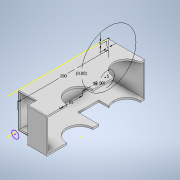
# Autodesk Inventor part: 차체 뚜껑
Saved by Autodesk Inventor 2021 (Build 250183000, 183)
## iProperties
Created: 2022-09-27
Part Number: 차체 뚜껑
Material: 일반
Document SubType Name: Modeling
Designer: SW2151
Density: 1 g/cm^3
Appearance: 기본값
Author: SW2151
Autodesk Inventor part; units mm, degrees
ref_plane "YZ Plane" through (0, 0, 0) normal (1, 0, 0) x (0, 1, 0)
ref_plane "XZ Plane" through (0, 0, 0) normal (0, 1, 0) x (-1, 0, 0)
ref_plane "XY Plane" through (0, 0, 0) normal (0, 0, 1) x (1, 0, 0)
sketch "스케치1" plane through (0, 0, 0) normal (0, 1, 0) x (-1, 0, 0)
  line L0 (4.1347, 105.7038) -> (-100.8653, 105.7038)
  line L1 (-100.8653, 105.7038) -> (-100.8653, -184.2962)
  line L2 (-100.8653, -184.2962) -> (4.1347, -184.2962)
  line L3 (4.1347, -184.2962) -> (4.1347, 105.7038)
  point P0 (0, 0)
  dimension "d0" = 105
  dimension "d1" = 290
  constraints: 8 end point, 2 parallel, 1 horizontal, 1 perpendicular
  measures "d0" distance of L2.end L1.end
  measures "d1" distance of L1.end L0.end
sketch "스케치2" plane through (0, 0, 0) normal (0, 1, 0) x (-1, 0, 0)
  point P0 (0, 0)
sketch "스케치3" plane through (0, 0, 0) normal (0, 1, 0) x (-1, 0, 0)
  point P0 (0, 0)
sketch "스케치4" plane through (0, 0, 0) normal (0, 1, 0) x (-1, 0, 0)
  point P0 (0, 0)
extrude "돌출1" add sketch "스케치1" along normal blind 100
sketch "스케치5" plane through (100.8653, 0, 105.7038) normal (1, 0, 0) x (0, 0, -1)
  line L0 (0, 0) -> (290, 0) projected
  line L1 (290, 0) -> (285, 0)
  line L2 (285, 0) -> (285, 5)
  line L3 (285, 5) -> (290, 5)
  line L4 (290, 5) -> (290, 0)
  line L5 (290, 0) -> (290, 100) projected
  line L6 (290, 100) -> (285, 100)
  line L7 (285, 100) -> (285, 95)
  line L8 (285, 95) -> (290, 95)
  line L9 (290, 95) -> (290, 100)
  line L10 (285, 5) -> (35, 5)
  line L11 (35, 5) -> (35, 95)
  line L12 (35, 95) -> (285, 95)
  line L13 (285, 95) -> (285, 5)
  point P0 (105.7038, 0)
  dimension "d4" = 5
  dimension "d5" = 5
  dimension "d6" = 5
  dimension "d7" = 5
  dimension "d8" = 250
  dimension "d9" = 90
  constraints: 24 end point, 6 parallel, 3 horizontal, 3 perpendicular
  measures "d4" distance of L2.end L3.end
  measures "d5" distance of L1.end L2.end
  measures "d6" distance of L8.end L7.end
  measures "d7" distance of L7.end L6.end
  measures "d8" distance of L11.end L12.end
  measures "d9" distance of L10.end L11.end
extrude "돌출2" cut sketch "스케치5" against normal blind 100 contours L10 L11 L12 L13
sketch "스케치6" plane through (100.8653, 0, 105.7038) normal (1, 0, 0) x (0, 0, -1)
  point P0 (105.7038, 0)
sketch "스케치7" plane through (100.8653, 0, 105.7038) normal (1, 0, 0) x (0, 0, -1)
  line L0 (285, 5) -> (35, 5) projected
  line L1 (35, 5) -> (11, 5)
  line L2 (11, 5) -> (11, 95)
  line L3 (11, 95) -> (35, 95)
  line L4 (35, 95) -> (35, 5)
  point P0 (105.7038, 0)
  dimension "d12" = 24
  constraints: 8 end point, 2 parallel, 1 horizontal, 1 perpendicular
  measures "d12" distance of L2.end L3.end
extrude "돌출3" cut sketch "스케치7" against normal blind 100
sketch "스케치8" plane through (-4.1347, 0, 105.7038) normal (0, 0, 1) x (1, 0, 0)
  circle A0 centre (22.6105, 17.0226) radius 10.2543
  point P0 (4.1347, 0)
  constraints: 1 centre point
sketch "스케치11" plane through (-4.1347, 0, -184.2962) normal (-1, 0, 0) x (0, 0, 1)
  point P0 (184.2962, 0)
sketch "스케치9" plane through (-4.1347, 0, -184.2962) normal (-1, 0, 0) x (0, 0, 1)
  line L0 (290, 100) -> (0, 100) projected
  line L1 (0, 100) -> (5, 100)
  line L2 (5, 100) -> (5, 95)
  line L3 (5, 95) -> (0, 95)
  line L4 (0, 95) -> (0, 100)
  line L5 (0, 0) -> (5, 0)
  line L6 (0, 0) -> (290, 0) projected
  line L7 (5, 0) -> (75, 0)
  line L8 (5, 0) -> (75, 0) construction
  line L9 (75, 0) -> (140, 0)
  line L10 (75, 0) -> (184.2962, 0)
  dimension "d15" = 5
  dimension "d16" = 5
  dimension "d17" = 5
  dimension "d18" = 70
  dimension "d19" = 0
  dimension "d20" = 65
  constraints: 18 end point, 3 horizontal, 2 collinear, 2 parallel, 2 point on line, 1 perpendicular
  measures "d15" distance of L2.end L3.end
  measures "d16" distance of L1.end L2.end
  measures "d17" distance of L5.start L5.end
  measures "d18" distance of L5.end L7.end
  measures "d19" distance between parallel lines of L7 L8
  measures "d20" distance of L7.end L9.end
sketch "스케치12" plane through (-4.1347, 0, -184.2962) normal (-1, 0, 0) x (0, 0, 1)
  point P0 (184.2962, 0)
sketch "스케치10" plane through (0, 0, 0) normal (0, -1, 0) x (1, 0, 0)
  point P0 (0, 0)
sketch "스케치13" plane through (-4.1347, 0, -184.2962) normal (-1, 0, 0) x (0, 0, 1)
  point P0 (184.2962, 0)
sketch "스케치14" plane through (0, 0, 0) normal (0, -1, 0) x (1, 0, 0)
  line L0 (-4.1347, -184.2962) -> (-4.1347, 105.7038) projected
  line L1 (-4.1347, -110.8863) -> (100.8653, -110.8863)
  line L2 (100.8653, 105.7038) -> (100.8653, -184.2962) projected
  line L3 (100.8653, -110.8863) -> (40.8653, -110.8863)
  line L4 (40.8653, -110.8863) -> (40.8653, -50.8863)
  line L5 (40.8653, -50.8863) -> (100.8653, -50.8863)
  line L6 (100.8653, -50.8863) -> (100.8653, -110.8863)
  point P0 (0, 0)
  dimension "d21" = 60
  dimension "d22" = 60
  constraints: 10 end point, 2 horizontal, 2 parallel, 2 point on line, 1 perpendicular
  measures "d21" distance of L4.end L5.end
  measures "d22" distance of L3.end L4.end
extrude "돌출4" cut sketch "스케치14" against normal blind 80
sketch "스케치15" plane through (0, 0, 0) normal (0, -1, 0) x (1, 0, 0)
  line L0 (100.8653, -184.2962) -> (-4.1347, -184.2962) projected
  line L1 (100.8653, -184.2962) -> (100.8653, -169.2962)
  line L2 (100.8653, -110.8863) -> (100.8653, -184.2962) projected
  line L3 (100.8653, -169.2962) -> (100.8653, -131.7962)
  circle A0 centre (100.8653, -131.7962) radius 37.5
  point P0 (0, 0)
  dimension "d25" = 15
  dimension "d26" = 37.5
  dimension "d27" = 75
  constraints: 4 end point, 2 point on line, 1 centre point, 1 coincident
  measures "d25" distance of L0.start L1.end
  measures "d26" distance of L1.end L3.end
  measures "d27" diameter of A0
extrude "돌출5" cut sketch "스케치15" against normal blind 80
sketch "스케치16" plane through (0, 0, 0) normal (0, -1, 0) x (1, 0, 0)
  arc A0 (69.7361, -110.8863) -> (100.8653, -169.2962) centre (100.8653, -131.7962) ccw projected
  line L0 (100.8653, -169.2962) -> (100.8653, -94.2962)
  line L1 (100.8653, 94.7038) -> (100.8653, -179.2962) projected
  line L2 (100.8653, -169.2962) -> (175.8653, -169.2962) construction
  line L3 (100.8653, -94.2962) -> (100.8653, -34.2962)
  line L4 (100.8653, -34.2962) -> (100.8653, 3.2038)
  circle A1 centre (100.8653, 3.2038) radius 37.5
  point P0 (0, 0)
  point P1 (100.8653, 40.7038)
  dimension "d30" = 75
  dimension "d31" = 90
  dimension "d32" = 60
  dimension "d33" = 37.5
  dimension "d34" = 180
  dimension "d35" = 75
  constraints: 8 end point, 2 collinear, 1 centre point, 1 coincident, 1 horizontal, 1 perpendicular, 1 point on line
  measures "d30" distance of L0.start L0.end
  measures "d31" angle of L2 L0
  measures "d32" distance of L0.end L3.end
  measures "d33" distance of L3.end L4.end
  measures "d34" angle of L4 L3
  measures "d35" diameter of A1
extrude "돌출6" cut sketch "스케치16" against normal blind 8300 contours L1 A1 picked at (87.6481, -17.8312)
sketch "스케치17" plane through (0, 0, 0) normal (0, -1, 0) x (1, 0, 0)
  line L0 (100.8653, -34.2962) -> (100.8653, -184.2962) projected
  line L1 (100.8653, -184.2962) -> (100.8653, -169.0212)
  line L2 (100.8653, -169.0212) -> (100.8653, -131.5212)
  circle A0 centre (100.8653, -131.5212) radius 37.5
  point P0 (0, 0)
  point P1 (100.8653, -94.0212)
  dimension "d38" = 15.275
  dimension "d39" = 37.5
  dimension "d40" = 75
  constraints: 4 end point, 2 point on line, 1 centre point, 1 coincident
  measures "d38" distance of L0.end L1.end
  measures "d39" distance of L1.end L2.end
  measures "d40" diameter of A0
extrude "돌출7" cut sketch "스케치17" against normal blind 8300 contours L0 A0 picked at (87.6481, -152.5562)
sketch "스케치18" plane through (-4.1347, 0, -184.2962) normal (-1, 0, 0) x (0, 0, 1)
  line L0 (0, 0) -> (0, 100) projected
  line L1 (0, 50) -> (260, 50)
  line L2 (0, 50) -> (260, 50) construction
  point P0 (184.2962, 0)
  dimension "d43" = 260
  dimension "d44" = 0
  constraints: 4 end point, 2 horizontal, 1 collinear, 1 midpoint
  measures "d43" distance of L1.start L1.end
  measures "d44" distance between parallel lines of L1 L2
sketch "스케치19" plane through (-4.1347, 0, -184.2962) normal (-1, 0, 0) x (0, 0, 1)
  line L0 (259.9404, 50.2138) -> (259.9404, 99.3471)
  line L1 (259.9404, 99.3471) -> (259.9404, 100)
  line L2 (290, 100) -> (225, 100) projected
  line L3 (290, 0) -> (225, 0) projected
  line L4 (259.9404, 100) -> (290, 100)
  line L5 (290, 100) -> (290, 0)
  line L6 (290, 0) -> (259.9404, 0)
  line L7 (259.9404, 0) -> (259.9404, 100)
  point P0 (184.2962, 0)
  constraints: 12 end point, 2 parallel, 2 vertical, 1 horizontal, 1 perpendicular, 1 point on line
extrude "돌출8" cut sketch "스케치19" against normal blind 50
sketch "스케치24" plane through (100.8653, 0, -184.2962) normal (0, 0, -1) x (-1, 0, 0)
  line L0 (0, 0) -> (0, 5) projected
  line L1 (103, 100) -> (0, 100)
  line L2 (0, 100) -> (0, 0)
  line L3 (0, 0) -> (103, 0)
  line L4 (103, 0) -> (103, 100)
  point P0 (100.8653, 0)
  constraints: 8 end point, 2 parallel, 1 horizontal, 1 perpendicular
extrude "돌출12" cut sketch "스케치24" against normal blind 3
sketch "스케치26" plane through (100.8653, 0, 105.7038) normal (0, 0, 1) x (1, 0, 0)
  line L0 (-55, 100) -> (0, 100) projected
  line L1 (0, 5) -> (0, 0) projected
  line L2 (-55, 100) -> (0, 100)
  line L3 (0, 100) -> (0, 0)
  line L4 (0, 0) -> (-55, 0)
  line L5 (-55, 0) -> (-55, 100)
  point P0 (-100.8653, 0)
  constraints: 8 end point, 2 parallel, 1 horizontal, 1 perpendicular
extrude "돌출14" cut sketch "스케치26" against normal blind 7
fillet "모깎기7" radius 2 14 edges at (45.8653, 50, 98.7038) (73.3653, 100, 98.7038) (73.3653, 0, 98.7038) (45.8653, 50, 94.7038) (45.8653, 5, 85.1739) (23.3653, 5, 75.6441) (0.8653, 50, 75.6441) (-4.1347, 50, 75.6441) (23.3653, 95, 75.6441) (20.8653, 100, 75.6441) (20.8653, 0, 75.6441) (45.8653, 95, 85.1739) (45.8653, 100, 87.1739) (45.8653, 0, 87.1739)
sketch "스케치20" plane through (-4.1347, 98, -184.2962) normal (-1, 0, 0) x (0, 0, 1)
  line L0 (99.3624, -73.1284) -> (157.5725, -73.1284)
  line L1 (157.5725, -73.1284) -> (157.5725, -19.1517)
  line L2 (157.5725, -19.1517) -> (99.3624, -19.1517)
  line L3 (99.3624, -19.1517) -> (99.3624, -73.1284)
  point P0 (184.2962, -98)
  constraints: 8 end point, 2 parallel, 1 horizontal, 1 perpendicular
sketch "스케치21" plane through (-14.1347, 98, -184.2962) normal (-1, 0, 0) x (0, 0, 1)
  line L0 (87.1912, -87.9455) -> (166.5686, -87.9455)
  line L1 (166.5686, -87.9455) -> (166.5686, -6.4514)
  line L2 (166.5686, -6.4514) -> (87.1912, -6.4514)
  line L3 (87.1912, -6.4514) -> (87.1912, -87.9455)
  line L4 (87.1912, -87.9455) -> (166.5686, -6.4514) construction
  line L5 (166.5686, -87.9455) -> (87.1912, -6.4514) construction
  point P0 (184.2962, -98)
  point P1 (126.8799, -47.1984)
  constraints: 12 end point, 2 midpoint, 2 parallel, 1 horizontal, 1 perpendicular
sketch "스케치22" plane through (-24.1347, 98, -184.2962) normal (-1, 0, 0) x (0, 0, 1)
  line L0 (162.3351, -80.537) -> (95.6581, -80.537)
  line L1 (95.6581, -80.537) -> (95.6581, -12.8016)
  line L2 (95.6581, -12.8016) -> (162.3351, -12.8016)
  line L3 (162.3351, -12.8016) -> (162.3351, -80.537)
  line L4 (162.3351, -80.537) -> (95.6581, -12.8016) construction
  line L5 (95.6581, -80.537) -> (162.3351, -12.8016) construction
  point P0 (184.2962, -98)
  point P1 (128.9966, -46.6693)
  constraints: 12 end point, 2 midpoint, 2 parallel, 1 horizontal, 1 perpendicular
